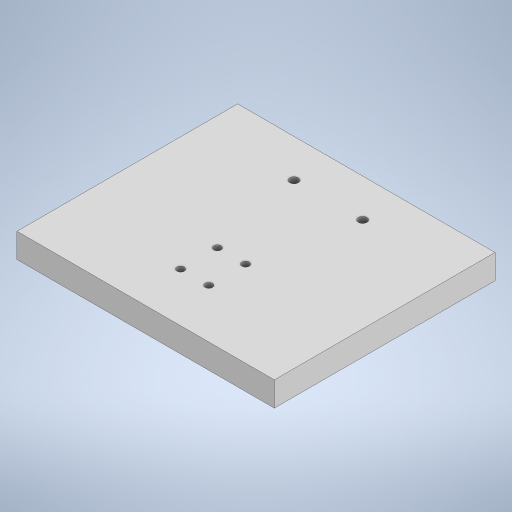
# Autodesk Inventor part: base_front
Saved by Autodesk Inventor 2023 (Build 270158000, 158)
## iProperties
Created: 2022-10-20
Part Number: base_front
Material: Genérico
Document SubType Name: Modeling
Designer: inigo
Density: 1 g/cm^3
Appearance: Valor por defecto
Author: inigo
Autodesk Inventor part; units mm, degrees
ref_plane "YZ Plane" through (0, 0, 0) normal (1, 0, 0) x (0, 1, 0)
ref_plane "XZ Plane" through (0, 0, 0) normal (0, 1, 0) x (-1, 0, 0)
ref_plane "XY Plane" through (0, 0, 0) normal (0, 0, 1) x (1, 0, 0)
sketch "Boceto1" plane through (0, 0, 0) normal (0, 1, 0) x (-1, 0, 0)
  line L0 (105, 90) -> (-105, 90)
  line L1 (-105, 90) -> (-105, -90)
  line L2 (-105, -90) -> (105, -90)
  line L3 (105, -90) -> (105, 90)
  line L4 (105, 90) -> (-105, -90) construction
  line L5 (-105, 90) -> (105, -90) construction
  point P0 (0, 0)
  dimension "d0" = 210
  dimension "d1" = 180
  constraints: 12 end point, 2 midpoint, 2 parallel, 1 horizontal, 1 perpendicular
  measures "d0" distance of L2.end L1.end
  measures "d1" distance of L1.end L0.end
extrude "Extrusión1" add sketch "Boceto1" along normal blind 20
sketch "Boceto2" plane through (0, 20, 0) normal (0, 1, 0) x (1, 0, 0)
  line L0 (-105.0239, -70) -> (104.9761, -70)
  line L1 (-105.0239, -70) -> (104.9761, -70)
  circle A0 centre (-11.5239, -50) radius 3
  circle A1 centre (11.4761, -50) radius 3
  circle A2 centre (-11.5239, -20) radius 3
  circle A3 centre (11.4761, -20) radius 3
  line L2 (-105, -90) -> (105, -90) projected
  circle A4 centre (28, 59) radius 3.5
  circle A5 centre (-28, 59) radius 3.5
  line L3 (105, 90) -> (-105, 90) projected
  line L4 (0, 90) -> (0, 53.0386)
  point P0 (0, 0)
  point P1 (0, -225)
  point P2 (0, -225)
  dimension "d4" = 20
  dimension "d5" = 20
  dimension "d6" = 30
  dimension "d7" = 30
  dimension "d8" = 20
  dimension "d9" = 7
  dimension "d11" = 7
  dimension "d12" = 31
  dimension "d13" = 31
  dimension "d14" = 28
  dimension "d15" = 28
  constraints: 6 centre point, 6 end point, 1 collinear, 1 midpoint, 1 vertical
  measures "d4" distance from line of L0 A0.centre
  measures "d5" distance from line of A1.centre L0
  measures "d6" distance between centres of A3 A1
  measures "d7" distance of A2.centre A0.centre
  measures "d8" distance between parallel lines of L2 L0
  measures "d9" diameter of A4
  measures "d11" diameter of A5
  measures "d12" distance from line of A5.centre L3
  measures "d13" distance from line of L3 A4.centre
  measures "d14" distance from line of L4 A4.centre
  measures "d15" distance from line of L4 A5.centre
extrude "Extrusión2" cut sketch "Boceto2" against normal blind 20
